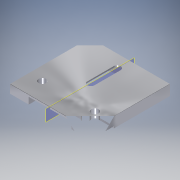
# Autodesk Inventor part: Portal-Column-v2-Column
Saved by Autodesk Inventor 2016 (Build 200138000, 138)
## iProperties
Created: 2015-10-23
Part Number: Portal-Column-v2-Column
Material: Aluminum 6061
Document SubType Name: Modeling
Designer: as
Density: 2.7 g/cm^3
Appearance: Aluminum - Flat
Mass: 40.6429 g
Surface Area: 94.8855 cm^2
Volume: 15.0529 cm^3
Author: as
Autodesk Inventor part; units mm, degrees
ref_plane "YZ Plane" through (0, 0, 0) normal (1, 0, 0) x (0, 1, 0)
ref_plane "XZ Plane" through (0, 0, 0) normal (0, 1, 0) x (-1, 0, 0)
ref_plane "XY Plane" through (0, 0, 0) normal (0, 0, 1) x (1, 0, 0)
sketch "Sketch1" plane through (0, 0, 0) normal (0, 0, 1) x (1, 0, 0)
  line L0 (0, 0) -> (60, 0)
  line L1 (60, 0) -> (60, -60)
  line L2 (60, -60) -> (0, -60)
  line L3 (0, -60) -> (0, 0)
  dimension "d0" = 60
  dimension "d1" = 60
  constraints: 8 end point, 2 parallel, 1 horizontal, 1 perpendicular
  measures "d0" distance of L1.end L2.end
  measures "d1" distance of L0.end L1.end
extrude "Extrusion1" add sketch "Sketch1" along normal blind 8
move faces "Move1" translate (0, 50, 0) faces at (20, 0, 2.6667)
move faces "Move2" translate (0, 50, 0) faces at (40, -60, 2.6667)
sketch "Sketch2" plane through (0, 0, 8) normal (0, 0, 1) x (1, 0, 0)
  point P0 (49.7, 4)
hole "Hole1" at (49.7, 4, 8) direction (0, 0, -1) diameter 5.5 depth 8
ref_plane "Work Plane1" through (30, 50, 0) normal (-1, 0, 0) x (0, 0, 1)
mirror "Mirror1" about plane through (30, 50, 0) normal (-1, 0, 0) of "Hole1"
sketch "Sketch3" plane through (0, 50, 0) normal (0, 1, 0) x (1, 0, 0)
  line L0 (0, 0) -> (60, 0) construction
  line L1 (10, 0) -> (10, -4) construction
  line L2 (10, -4) -> (10, -8) construction
  line L3 (60, -8) -> (0, -8) construction
  line L4 (10, -4) -> (0, -4) construction
  line L5 (0, 0) -> (0, -8) construction
  dimension "d17" = 10
  constraints: 6 end point, 2 point on line, 2 vertical, 1 coincident, 1 collinear, 1 midpoint
  measures "d17" distance of L1.end L4.end
hole "Hole3" at (10, 50, 4) direction (0, -1, 0) diameter 4 depth 15 tip angle 118
mirror "Mirror2" about plane through (30, 50, 0) normal (-1, 0, 0) of "Hole3"
sketch "Sketch4" plane through (0, 0, 0) normal (0, 0, -1) x (-1, 0, 0)
  circle A0 centre (-10.3, 4) radius 2.75 projected
  circle A1 centre (-49.7, 4) radius 2.75 projected
  line L0 (0, 50) -> (-60, 50) projected
  line L1 (-60, 50) -> (-60, -10) projected
  line L2 (-60, -10) -> (0, -10) projected
  line L3 (0, -10) -> (0, 50) projected
  line L4 (-60, -10) -> (-60, 50) projected
  line L5 (-39.4, 0) -> (-60, 0)
  line L6 (-60, 0) -> (-60, 8)
  line L7 (-60, 8) -> (-39.4, 8)
  line L8 (-39.4, 0) -> (-60, 8) construction
  line L9 (-60, 0) -> (-39.4, 8) construction
  line L10 (-39.4, 8) -> (-30, 8)
  line L11 (-30, 8) -> (-30, 0)
  line L12 (-30, 0) -> (-39.4, 0)
  line L13 (-48, 35) -> (-48, 16.6)
  arc A2 (-44.4772, 40.9525) -> (-48, 35) centre (-41.2097, 35) ccw
  arc A3 (-30, 45) -> (-44.4772, 40.9525) centre (-28.5718, 11.977) ccw
  arc A4 (-48, 16.6) -> (-39.4, 8) centre (-39.4, 16.6) ccw
  line L14 (-39.4, 8) -> (-39.4, 16.6) construction
  line L15 (-48, 16.6) -> (-39.4, 16.6) construction
  line L16 (-60, -10) -> (0, -10)
  line L17 (0, -10) -> (0, 0)
  line L18 (0, 0) -> (-60, 0)
  line L19 (-60, 0) -> (-60, -10)
  line L20 (-30, 45) -> (-30, 8)
  dimension "d27" = 8
  dimension "d28" = 90
  constraints: 32 end point, 6 point on circle, 4 parallel, 4 perpendicular, 3 centre point, 3 horizontal, 3 tangent, 2 midpoint, 1 point on line, 1 vertical
  measures "d27" distance of L5.end L6.end
  measures "d28" angle of L15 L14
extrude "Extrusion2" cut sketch "Sketch4" against normal blind 7 contours A4 L13 A2 A3 L20 L10
mirror "Mirror3" about plane through (30, 50, 0) normal (-1, 0, 0) of "Extrusion2"
sketch "Sketch5" plane through (0, 0, 0) normal (0, 0, -1) x (-1, 0, 0)
  line L0 (-73.1915, 8) -> (-27.8, 8)
  line L1 (-73.1915, 8) -> (9.8865, 8)
  line L2 (9.8865, 8) -> (9.8865, -10)
  line L3 (9.8865, -10) -> (-73.1915, -10)
  line L4 (-73.1915, -10) -> (-73.1915, 8)
  point P0 (0, 0)
  constraints: 10 end point, 2 parallel, 1 horizontal, 1 perpendicular
extrude "Extrusion3" cut sketch "Sketch5" against normal blind 1.5
fillet "Fillet1" radius 1.5 2 edges at (39.4, 8, 0.75) (20.6, 8, 0.75)
sketch "Sketch6" plane through (0, 0, 1.5) normal (0, 0, -1) x (-1, 0, 0)
  line L0 (-46, -20) -> (-14, -20)
  line L1 (-14, -20) -> (-14, 0)
  line L2 (-14, 0) -> (-46, 0)
  line L3 (-46, 0) -> (-46, -20)
  line L4 (0, -10) -> (-60, -10) projected
  line L5 (-46, -20) -> (-14, 0) construction
  line L6 (-14, -20) -> (-46, 0) construction
  point P0 (0, 0)
  point P1 (-30, -10)
  point P2 (-32.2, -10)
  dimension "d37" = 32
  constraints: 12 end point, 3 midpoint, 2 parallel, 1 horizontal, 1 perpendicular
  measures "d37" distance of L2.end L1.end
extrude "Extrusion4" cut sketch "Sketch6" against normal blind 5
fillet "Fillet2" radius 3.5 2 edges at (14, 0, 4) (46, 0, 4)
sketch "Sketch7" plane through (0, 0, 7) normal (0, 0, -1) x (-1, 0, 0)
  line L0 (-30, 43.0622) -> (-30, 18.0622) construction
  line L1 (-32.6, 40.4622) -> (-32.6, 20.6622)
  line L2 (-27.4, 20.6622) -> (-27.4, 40.4622)
  arc A0 (-27.4, 40.4622) -> (-32.6, 40.4622) centre (-30, 40.4622) ccw
  arc A1 (-32.6, 20.6622) -> (-27.4, 20.6622) centre (-30, 20.6622) ccw
  point P0 (0, 0)
  point P1 (-30, 30.5622)
  dimension "d41" = 25
  dimension "d42" = 5.2
  constraints: 8 end point, 6 point on circle, 4 tangent, 2 centre point, 2 point on line, 1 midpoint, 1 parallel, 1 vertical
  measures "d41" distance of L0.start L0.end
  measures "d42" diameter of A1
extrude "Extrusion5" cut sketch "Sketch7" against normal through all
chamfer "Chamfer2" distance 0.1 angle 45 14 edges at (30, 50, 0) (60, 50, 4) (30, 50, 8) (0, 50, 4) (60, 29, 0) (60, 20, 8) (0, 29, 0) (0, 20, 8) (0, -10, 4.75) (30, -10, 8) (60, -10, 4.75) (30, -10, 6.5) (7, -10, 1.5) (53, -10, 1.5)
body "Solid1"
